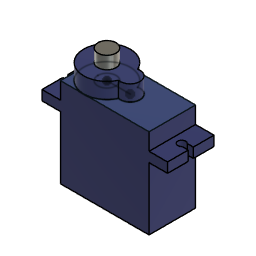
Rotating_Disc (Autodesk Fusion 360 archive; units mm, degrees)
design "Motor"
Autodesk Fusion 360 part; units mm, degrees
sketch "Sketch1" plane through (0, 0, 0) normal (0, 0, 1) x (1, 0, 0)
  line L0 (11.25, 5.9) -> (-11.25, 5.9)
  line L1 (-11.25, 5.9) -> (-11.25, -5.9)
  line L2 (-11.25, -5.9) -> (11.25, -5.9)
  line L3 (11.25, -5.9) -> (11.25, 5.9)
  line L4 (11.25, 5.9) -> (-11.25, -5.9) construction
  line L5 (-11.25, 5.9) -> (11.25, -5.9) construction
  dimension "d1" = 22.5
  dimension "d2" = 11.8
  constraint horizontal L0
  constraint perpendicular L0 L1
  constraint parallel L0 L2
  constraint parallel L1 L3
  constraint coincident L4 origin
  constraint coincident L5 origin
  measures "d1" distance of L1.end L2.end
  measures "d2" distance of L0.end L1.end
extrude "Extrude1" add sketch "Sketch1" along normal blind 22.7 makes body 1
sketch "Sketch2" plane through (11.25, 0, 0) normal (1, 0, 0) x (0, 1, 0)
  line L0 (-5.9, 0) -> (5.9, 0)
  line L1 (5.9, 0) -> (5.9, 22.7)
  line L2 (5.9, 22.7) -> (-5.9, 22.7)
  line L3 (-5.9, 22.7) -> (-5.9, 0)
  line L4 (5.9, 22.7) -> (5.9, 18.4)
  line L5 (5.9, 18.4) -> (-5.9, 18.4)
  line L6 (-5.9, 18.4) -> (-5.9, 15.9)
  line L7 (-5.9, 15.9) -> (5.9, 15.9)
  line L8 (5.9, 15.9) -> (5.9, 18.4)
  dimension "d5" = 4.3
  dimension "d6" = 2.5
  constraint coincident L1.end L2.start
  constraint perpendicular L2 L4
  constraint horizontal L5
  constraint vertical L6
  constraint horizontal L7
  constraint vertical L8
  measures "d5" distance of L1.end L4.end
  measures "d6" distance of L4.end L7.end
extrude "Extrude2" add sketch "Sketch2" along normal blind 4.7 contours L1 L3 L5 L6 L7 L8 bodies 1
sketch "Sketch3" plane through (0, 0, 18.4) normal (0, 0, 1) x (-1, 0, 0)
  line L0 (-11.25, -5.9) -> (-11.25, 5.9)
  line L1 (-11.25, 5.9) -> (-15.95, 5.9)
  line L2 (-15.95, 5.9) -> (-15.95, -5.9)
  line L3 (-15.95, -5.9) -> (-11.25, -5.9)
  line L4 (-15.95, -5.9) -> (-15.95, 0)
  line L5 (-15.95, 0) -> (-13.65, 0)
  line L6 (-14.4099, -0.65) -> (-15.95, -0.65)
  line L7 (-14.4099, 0.65) -> (-15.95, 0.65)
  arc A0 (-14.4099, -0.65) -> (-14.4099, 0.65) centre (-13.65, 0) ccw
  dimension "d9" = 2.3
  dimension "d10" = 2
  dimension "d12" = 0.65
  constraint coincident L2.end L3.start
  constraint midpoint L2 L4.end
  constraint perpendicular L2 L5
  constraint coincident L5.end A0.centre
  constraint horizontal L6
  constraint coincident L2 L6.end
  constraint symmetric L5 L6.start L7.start
  constraint symmetric L5 L6.end L7.end
  measures "d9" distance of L4.end L5.end
  measures "d10" diameter of A0
  measures "d12" distance of L5 L6
extrude "Extrude3" cut sketch "Sketch3" against normal blind 3 contours L2 L4 L6 L7 A0 bodies 1
mirror "Mirror1" about plane through (0, 0, 0) normal (1, 0, 0) of bodies 1 merged
sketch "Sketch4" plane through (0, 0, 22.7) normal (0, 0, 1) x (-1, 0, 0)
  line L0 (-11.25, 5.9) -> (-11.25, -5.9)
  line L1 (-11.25, -5.9) -> (11.25, -5.9)
  line L2 (11.25, -5.9) -> (11.25, 5.9)
  line L3 (11.25, 5.9) -> (-11.25, 5.9)
  circle A0 centre (5.35, 0) radius 2.3
  arc A1 (-0.0203, 2.4432) -> (-0.0203, -2.4432) centre (-0.55, 0) ccw
  arc A2 (-0.0203, -2.4432) -> (-0.0203, 2.4432) centre (5.35, 0) ccw
  line L4 (5.35, 0) -> (-0.55, 0)
  dimension "d17" = 11.8
  dimension "d18" = 4.6
  dimension "d19" = 5
  constraint tangent L2 A2
  constraint tangent L1 A2
  constraint concentric A0 A2
  constraint coincident A1.centre A2
  constraint coincident A0.centre A2.centre
  constraint coincident A1.centre L4.end
  constraint horizontal L4
  measures "d17" diameter of A2
  measures "d18" diameter of A0
  measures "d19" diameter of A1
extrude "Extrude4" add sketch "Sketch4" along normal blind 4 contours A1 A2 bodies 1
sketch "Sketch5" plane through (0, 0, 0) normal (0, 0, 1) x (1, 0, 0)
  circle A0 centre (20, 0) radius 2.3
  dimension "d24" = 4.6
  measures "d24" diameter of A0
extrude "Extrude6" add sketch "Sketch5" along normal blind 3.2 separate body makes body 2
copy_body "Body->Comp1" bodies 2 removing the originals makes body 3 in component "Component"
component "Component" placed x (1, 0, 0) y (0, -1, 0) z (0, 0, -1) at (-25.35, 0, 29.9)
